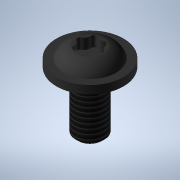
# Autodesk Inventor part: 0000-00082819_P2
Saved by Autodesk Inventor 2021 (Build 250183000, 183)
## iProperties
Created: 2025-07-29
Part Number: 0000-00082819_P2
Material: Generic
Catalog Web Link: www.cadenas.de
Description: Schrauben fur Flanschplatte KL 2.0-Schrauben fur Flanschplatte KL 2.0
Vendor: RITTAL
Document SubType Name: Modeling
Designer: psAdmin
Manufacturer: RITTAL
Mass: 0.399764 g
Surface Area: 4.55483 cm^2
Volume: 0.399764 cm^3
Density: 1 g/cm^3
Appearance: PSOLRGB-176-176-176
Category: PARTsolutions
Company: RITTAL
Title: 0000-00082819_P2
Author: Cadenas PARTsolutions
Comments: Schrauben fur Flanschplatte KL 2.0
PSOL_IDENT_0: {$CADENAS_DATA/23d-libs/rittal/schaltschranksys/kleingeh/parts_kl_2_0/schrauben_flanschplatte_kl_2_0
PSOL_IDENT_1: .prj},200 {VTYP=3D},{NB=0000-00082819_P2},{LINA=0000-00082819_P2},{NN=Schrauben fur Flanschplatte KL
PSOL_IDENT_2: 2.0},{DATE=27.11.2019 12:11:25},{GEOMDATE=02.09.2019 05:43:46},{VERSION=},{LINEID=10},{WBVAR=},{WBN
PSOL_IDENT_3: UMERIC=}  {NB=0000-00082819_P2},{LINA=0000-00082819_P2},{KT=DUMMY},{BEST=0000-00082819}
NB: 0000-00082819_P2
NN: Schrauben fur Flanschplatte KL 2.0
NT: Schrauben fur Flanschplatte KL 2.0
NBSYN: $BEST._P2
LINA: 0000-00082819_P2
CATALOG: Rittal
BEST: 0000-00082819
SUPPLIER: RITTAL
ARTICLENO: 0000-00082819_P2
BOMINFO: 0000-00082819_P2
CREATOR: CADENAS GmbH
Autodesk Inventor part; units mm, degrees
sketch "Sketch_3" plane through (0, 0, 0) normal (0, 0, 1) x (1, 0, 0)
  line L0 (0, -8.75) -> (0, 4.45)
  line L1 (0, 4.45) -> (2.3483, 4.45)
  arc A0 (4.4749, 2.65) -> (2.3483, 4.45) centre (1.695, 1.522) ccw
  line L2 (4.4749, 2.65) -> (5.75, 2.65)
  line L3 (5.75, 2.65) -> (5.75, 1.25)
  line L4 (5.75, 1.25) -> (2.5, 1.25)
  line L5 (2.5, 1.25) -> (2.5, -8.2595)
  line L6 (2.5, -8.2595) -> (2.0095, -8.75)
  line L7 (2.0095, -8.75) -> (0, -8.75)
  line L8 (0, -8.75) -> (0, 4.45)
  constraints: 18 end point, 2 point on circle, 1 centre point
revolve "Revolution1" add sketch "Sketch_3" angle 360 about axis through (0, -8.75, 0) along (0, -1, 0)
thread "Thread1" size "M5x0.8" class "6g" standard "ISO Metric profile" length 8.2595
sketch "Sketch_1" plane through (0, 4.45, 0) normal (0, 1, 0) x (1, 0, 0)
  arc A0 (-1.9719, 0.4486) -> (-1.9719, -0.4486) centre (-1.7511, 0) ccw
  arc A1 (-1.3744, -1.4834) -> (-1.9719, -0.4486) centre (-2.4461, -1.4123) ccw
  arc A2 (-1.3744, -1.4834) -> (-0.5974, -1.932) centre (-0.8755, -1.5165) ccw
  arc A3 (0.5974, -1.932) -> (-0.5974, -1.932) centre (0, -2.8245) ccw
  arc A4 (0.5974, -1.932) -> (1.3744, -1.4834) centre (0.8755, -1.5165) ccw
  arc A5 (1.9719, -0.4486) -> (1.3744, -1.4834) centre (2.4461, -1.4123) ccw
  arc A6 (1.9719, -0.4486) -> (1.9719, 0.4486) centre (1.7511, 0) ccw
  arc A7 (1.3744, 1.4834) -> (1.9719, 0.4486) centre (2.4461, 1.4123) ccw
  arc A8 (1.3744, 1.4834) -> (0.5974, 1.932) centre (0.8755, 1.5165) ccw
  arc A9 (-0.5974, 1.932) -> (0.5974, 1.932) centre (0, 2.8245) ccw
  arc A10 (-0.5974, 1.932) -> (-1.3744, 1.4834) centre (-0.8755, 1.5165) ccw
  arc A11 (-1.9719, 0.4486) -> (-1.3744, 1.4834) centre (-2.4461, 1.4123) ccw
  constraints: 24 point on circle, 12 centre point
extrude "Extrusion1" cut sketch "Sketch_1" against normal blind 1.8
ref_plane "Bolt_XY" through (0, 1.25, 0) normal (0, 1, 0) x (1, 0, 0)
ref_plane "Bolt_YZ" through (0, 1.25, 0) normal (1, 0, 0) x (0, 0, -1)
ref_plane "Bolt_ZX" through (0, 1.25, 0) normal (0, 0, -1) x (0, 1, 0)
body "Solid1"
